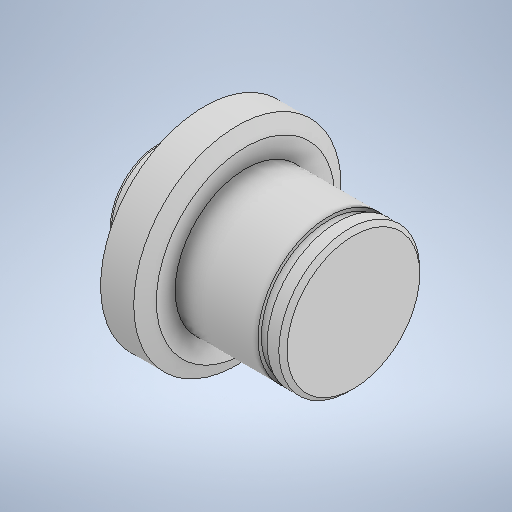
# Autodesk Inventor part: 26-10-208
Saved by Autodesk Inventor 2025.2 (Build 292293000, 293)
## iProperties
Created: 2024-11-29
Part Number: 26-10-208
Material: Generic
Document SubType Name: Modeling
Designer: Zvonko.Gabric
Density: 1 g/cm^3
Appearance: Default
Author: Zvonko.Gabric
Autodesk Inventor part; units mm, degrees
ref_plane "YZ Plane" through (0, 0, 0) normal (1, 0, 0) x (0, 1, 0)
ref_plane "XZ Plane" through (0, 0, 0) normal (0, 1, 0) x (-1, 0, 0)
ref_plane "XY Plane" through (0, 0, 0) normal (0, 0, 1) x (1, 0, 0)
sketch "Sketch1" plane through (0, 0, 0) normal (0, 1, 0) x (-1, 0, 0)
  line L0 (0, 0) -> (23.5, 0)
  line L1 (0.5, 8.5) -> (0, 8)
  line L2 (1.9, 8.5) -> (0.5, 8.5)
  line L3 (1.9, 8.1) -> (1.9, 8.5)
  line L4 (3, 8.1) -> (1.9, 8.1)
  line L5 (3, 8.5) -> (3, 8.1)
  line L6 (13, 8.5) -> (3, 8.5)
  line L7 (13, 10.7679) -> (13, 8.5)
  line L8 (14, 12.5) -> (13, 10.7679)
  line L9 (18, 12.5) -> (14, 12.5)
  line L10 (18, 6) -> (18, 12.5)
  line L11 (23.2, 6) -> (18, 6)
  line L12 (23.5, 5.8268) -> (23.2, 6)
  line L13 (23.5, 0) -> (23.5, 5.8268)
  line L14 (0, 0) -> (23.5, 0)
  line L15 (0, 8) -> (0, 0)
  dimension "d0" = 0
  dimension "d1" = 5.8268
  dimension "d2" = 0.3464
  dimension "d3" = 120
  dimension "d4" = 6
  dimension "d5" = 5.2
  dimension "d6" = 6.5
  dimension "d7" = 4
  dimension "d8" = 2
  dimension "d9" = 120
  dimension "d10" = 10
  dimension "d11" = 8.5
  dimension "d12" = 2.2679
  dimension "d13" = 0.4
  dimension "d14" = 1.1
  dimension "d15" = 0.4
  dimension "d16" = 1.4
  dimension "d17" = 135
  dimension "d18" = 0.7071
  dimension "d19" = 8
  dimension "d20" = 23.5
  dimension "d21" = 135
  constraints: 32 end point
  measures "d0" distance of L0.start point (0, 0)
  measures "d1" distance of L0.end L12.start
  measures "d2" distance of L12.start L11.start
  measures "d3" angle of L13 L12
  measures "d4" distance between parallel lines of L0 L11
  measures "d5" distance of L11.start L10.start
  measures "d6" distance of L10.start L9.start
  measures "d7" distance of L9.start L8.start
  measures "d8" distance of L8.start L7.start
  measures "d9" angle of L9 L8
  measures "d10" distance of L6.start L5.start
  measures "d11" distance between parallel lines of L0 L6
  measures "d12" distance of L7.start L6.start
  measures "d13" distance of L5.start L4.start
  measures "d14" distance of L4.start L3.start
  measures "d15" distance of L3.start L2.start
  measures "d16" distance of L2.start L1.start
  measures "d17" angle of L2 L1
  measures "d18" distance of L1.start L1.end
  measures "d19" distance of L1.end L0.start
  measures "d20" distance between parallel lines of L13 L15
  measures "d21" angle of L1 L15
revolve "Revolution1" add sketch "Sketch1" angle 360 about axis through (0, 0, 0) along (-1, 0, 0)
body "Solid1"
